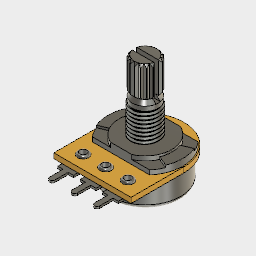
562 10K Potentiometer (Autodesk Fusion 360 design; units mm, degrees)
Autodesk Fusion 360 part; units mm, degrees
note: some values were not read from the file. Set by a fixed rule: which face or edge a step refers to.
sketch "Sketch2" plane through (0, 0, 0) normal (0, 0, 1) x (1, 0, 0)
  circle A0 centre (0, 0) radius 8.75
  line L0 (-8.75, 0) -> (8.75, 0)
  line L1 (8.75, 0) -> (8.75, -12)
  line L2 (8.75, -12) -> (-8.75, -12)
  line L3 (-8.75, -12) -> (-8.75, 0)
  circle A1 centre (-5.08, -9) radius 1.27
  circle A2 centre (-5.08, -9) radius 0.77
  circle A3 centre (0, -9) radius 0.77
  circle A4 centre (0, -9) radius 1.27
  circle A5 centre (5.08, -9) radius 0.77
  circle A6 centre (5.08, -9) radius 1.27
  dimension "d5" = 2.54
  dimension "d10" = 5.08
  dimension "d15" = 12
  dimension "d16" = 9
  dimension "d17" = 17.5
  dimension "d18" = 17.5
  dimension "d40" = 0.5
  dimension "d43" = 5.08
  dimension "d44" = 0
  measures "d5" diameter of A1
  measures "d10" distance of A0.centre A1.centre
  measures "d15" distance of L0.start L2.end
  measures "d16" distance of A0.centre A1.centre
  measures "d17" diameter of A0
  measures "d18" distance of L0.start L0.end
extrude "Extrude1" add sketch "Sketch2" against normal blind 1.2 contours A0 L0 | A0 L1 L2 L3 A4 | A0 L0 A4 | A0 A3 A4 | A0 A3 A4 | A1 | A6 makes body 1
extrude "Extrude9" add sketch "Sketch2" along normal blind 0.5 contours A0 A3 A4 | A0 A3 A4 | A1 | A6 bodies 1
fillet "Fillet2" radius 0.5 3 edges at (-6.2641, -9.4593, 0.5) (-1.1841, -9.4593, 0.5) (3.8959, -9.4593, 0.5) on bodies 1
sketch "Sketch4" plane through (0, 0, 0) normal (0, 0, 1) x (1, 0, 0)
  circle A0 centre (0, 0) radius 8.5
  line L0 (-10, 5.5) -> (10, 5.5)
  line L1 (10, 5.5) -> (10, -5.5)
  line L2 (10, -5.5) -> (-10, -5.5)
  line L3 (-10, -5.5) -> (-10, 5.5)
  circle A1 centre (0, 0) radius 6
  line L4 (0, 0) -> (11.8559, 4.9109)
  line L5 (0, 0) -> (15, 0) construction
  line L6 (0, 0) -> (-11.8559, 4.9109)
  line L7 (0, 0) -> (-11.8559, -4.9109)
  line L8 (0, 0) -> (11.8559, -4.9109)
  dimension "d19" = 17
  dimension "d20" = 11
  dimension "d21" = 12
  dimension "d27" = 22.5
  dimension "d29" = 360
  measures "d19" diameter of A0
  measures "d20" distance of L0.start L2.end
  measures "d21" diameter of A1
  measures "d27" angle of L4 L5
extrude "Extrude3" add sketch "Sketch4" along normal blind 1 separate body contours A0 A1 L4 L8 | A0 L0 A1 L4 | A0 L2 A1 L8 | L0 A1 L4 L6 | A1 L4 L8 | L2 A1 L7 L8 | A0 L0 A1 L6 | A1 L6 L7 | A0 L2 A1 L7 | A0 A1 L6 L7 makes body 2
extrude "Extrude4" add sketch "Sketch4" along normal blind 1 from surface at 1 contours L0 A1 L4 L6 | A1 L4 L8 | L2 A1 L7 L8 | A1 L6 L7 bodies 2
extrude "Extrude5" add sketch "Sketch4" along normal blind 0.5 from surface at 1 contours A0 A1 L4 L8 | A0 A1 L6 L7 bodies 2
sketch "Sketch5" plane through (0, 0, 2) normal (0, 0, 1) x (-1, 0, 0)
  line L0 (-2.3979, -5.5) -> (2.3979, -5.5)
  arc A0 (2.3979, -5.5) -> (2.3979, 5.5) centre (0, 0) ccw
  line L1 (2.3979, 5.5) -> (-2.3979, 5.5)
  arc A1 (-2.3979, 5.5) -> (-2.3979, -5.5) centre (0, 0) ccw
  circle A2 centre (0, 0) radius 3.3
  dimension "d33" = 6.6
  measures "d33" diameter of A2
extrude "Extrude6" add sketch "Sketch5" along normal blind 6.6 contours A2 bodies 2
sketch "Sketch6" plane through (0, 0, 8.6) normal (0, 0, 1) x (-1, 0, 0)
  circle A0 centre (0, 0) radius 3.3
  circle A1 centre (0, 0) radius 2.95
  dimension "d48" = 5.9
  measures "d48" diameter of A1
extrude "Extrude7" add sketch "Sketch6" along normal blind 1 separate body contours A1 makes body 3
extrude "Extrude8" add 1 faces at (1.3339, -0.3931, 9.6) along direction (0, 0, 1) blind 1 draft -45 on bodies 3 bodies 3
thread "Thread1" "ANSI Unified Screw Threads 0.25 1/4-32 UNEF 3A" major diameter 6.2738 minor diameter 5.4051 pitch 0.7937 angle 60 modelled right hand crest width 0.0992 on face at (-3.2959, 0.1645, 6.4) crest through (-3.1369, 0, 1.9504) on bodies 2
sketch "Sketch7" plane through (0, 0, 10.6) normal (0, 0, 1) x (-1, 0, 0)
  circle A0 centre (0, 0) radius 1.95
  circle A1 centre (0, 0) radius 3
  dimension "d49" = 6
  measures "d49" diameter of A1
extrude "Extrude10" add sketch "Sketch7" along normal blind 7 contours A0 | A1 bodies 3
sketch "Sketch8" plane through (0, 0, 17.6) normal (0, 0, 1) x (-1, 0, 0)
  circle A0 centre (0, 0) radius 3
  line L0 (0, -2.5) -> (-1, -3.5)
  line L1 (-1, -3.5) -> (1, -3.5)
  line L2 (1, -3.5) -> (0, -2.5)
  line L3 (-3.5, 0.5) -> (3.5, 0.5)
  line L4 (3.5, 0.5) -> (3.5, -0.5)
  line L5 (3.5, -0.5) -> (-3.5, -0.5)
  line L6 (-3.5, -0.5) -> (-3.5, 0.5)
  line L7 (-3.5, 0.5) -> (3.5, -0.5) construction
  line L8 (3.5, 0.5) -> (-3.5, -0.5) construction
  dimension "d52" = 1
  dimension "d53" = 7
  dimension "d54" = 1
  dimension "d62" = 2.5
  measures "d52" distance of L0.start L1
  measures "d53" distance of L4.end L5.end
  measures "d54" distance of L3.end L4.end
  measures "d62" distance of L0.start A0.centre
chamfer "Chamfer1" distance 0.5 angle 45 3 edges at (2.797, 1.0848, 17.6) (2.797, 1.0848, 17.6) (2.797, 1.0848, 10.6) on bodies 3
extrude "Extrude12" cut sketch "Sketch8" against normal up to surface (7 mm away) contours A0 L0 L2 bodies 3
pattern_circular "C-Pattern1" count 18 over 360 about axis through (0, 0, 17.6) along (0, 0, 1) of "Extrude12"
extrude "Extrude13" cut sketch "Sketch8" against normal blind 8 contours A0 L3 L5 bodies 3
sketch "Sketch9" plane through (0, 0, 0) normal (0, 0, 1) x (1, 0, 0)
  circle A0 centre (0, 0) radius 8
  dimension "d65" = 16
  measures "d65" diameter of A0
extrude "Extrude14" add sketch "Sketch9" against normal blind 6 from surface at -1.2 separate body makes body 4
fillet "Fillet3" radius 1 1 edges at (-7.4586, 2.8929, -7.2) on bodies 4
shell "Shell1" thickness 1 removed faces 1 at (-2.0217, -2.2578, -1.2) on bodies 4
sketch "Sketch10" plane through (0, 0, 0) normal (0, 1, 0) x (1, 0, 0)
  line L0 (-5, 0.5) -> (4.995, 0.5)
  line L1 (4.995, 0.5) -> (4.995, 2.1959)
  line L2 (4.995, 2.1959) -> (-5, 2.1959)
  line L3 (-5, 2.1959) -> (-5, 0.5)
extrude "Extrude15" cut sketch "Sketch10" against normal blind 11 bodies 4
sketch "Sketch11" plane through (0, 0, -1.2) normal (0, 0, -1) x (1, 0, 0)
  circle A0 centre (5.08, 9) radius 0.77
  circle A1 centre (-5.08, 9) radius 0.77
  circle A2 centre (0, 9) radius 0.77
  arc A3 (-8.75, 0) -> (8.75, 0) centre (0, 0) ccw
  line L0 (8.75, 0) -> (8.75, 12)
  line L1 (8.75, 12) -> (-8.75, 12)
  line L2 (-8.75, 12) -> (-8.75, 0)
  line L3 (6.88, 13) -> (6.88, 9)
  arc A4 (3.28, 9) -> (6.88, 9) centre (5.08, 9) ccw
  line L4 (3.28, 9) -> (3.28, 13)
  line L5 (3.28, 13) -> (6.88, 13)
  line L6 (5.68, 9) -> (5.68, 16)
  arc A5 (5.68, 16) -> (4.48, 16) centre (5.08, 16) ccw
  line L7 (4.48, 16) -> (4.48, 9)
  arc A6 (4.48, 9) -> (5.68, 9) centre (5.08, 9) ccw
  line L8 (5.08, 9) -> (5.08, 16) construction
  dimension "d73" = 3.6
  dimension "d74" = 4
  dimension "d75" = 1.2
  dimension "d82" = 3
  measures "d73" distance of L3.start L4.end
  measures "d74" distance of A0.centre L5
  measures "d75" diameter of A5
  measures "d82" distance of L5 A5.centre
extrude "Extrude16" add sketch "Sketch11" along normal blind 0.5 separate body contours A0 L1 L3 A4 L4 L6 L7 | A0 L1 L6 L7 | L1 L3 L5 L6 | L1 L5 L6 L7 | L1 L4 L5 L7 | L5 L6 A5 L7 makes body 5
pattern_linear "R-Pattern1" count 3 spacing 5.08 along (-1, 0, 0) of "Extrude16" makes body 6 at (-0.8381, -11.5872, -1.2) makes body 7 at (-5.9181, -11.5872, -1.2)
